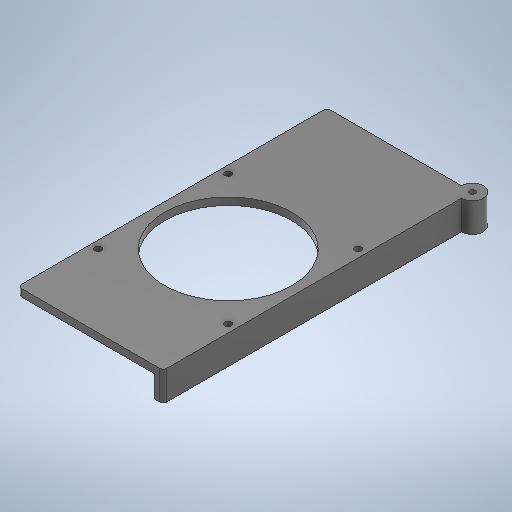
# Autodesk Inventor part: Power Box (12V) Cover
Saved by Autodesk Inventor 2026.2 (Build 302298010, 298A)
## iProperties
Created: 2026-05-26
Part Number: Power Box (12V) Cover
Material: ABS Plastic
Document SubType Name: Modeling
Designer: chanh
Density: 1.06 g/cm^3
Appearance: Smooth - White
Author: chanh
Autodesk Inventor part; units mm, degrees
ref_plane "YZ Plane" through (0, 0, 0) normal (1, 0, 0) x (0, 1, 0)
ref_plane "XZ Plane" through (0, 0, 0) normal (0, 1, 0) x (-1, 0, 0)
ref_plane "XY Plane" through (0, 0, 0) normal (0, 0, 1) x (1, 0, 0)
sketch "Sketch1" plane through (0, 0, 0) normal (0, 1, 0) x (-1, 0, 0)
  line L0 (40, 85) -> (-40, 85)
  line L1 (-40, 85) -> (-40, -85)
  line L2 (-40, -85) -> (40, -85)
  line L3 (40, -85) -> (40, 85)
  line L4 (40, 85) -> (-40, -85) construction
  line L5 (-40, 85) -> (40, -85) construction
  circle A0 centre (-40, -85) radius 6
  point P0 (0, 0)
  point P1 (-40, -79)
  point P2 (-34, -85)
  dimension "d0" = 80
  dimension "d1" = 170
  dimension "d2" = 12
  constraints: 12 end point, 2 midpoint, 2 parallel, 1 centre point, 1 coincident, 1 horizontal, 1 perpendicular
  measures "d0" distance of L2.end L1.end
  measures "d1" distance of L0.end L1.end
  measures "d2" diameter of A0
extrude "Extrusion1" add sketch "Sketch1" along normal blind 4
sketch "Sketch2" plane through (0, 0, 0) normal (0, -1, 0) x (1, 0, 0)
  line L0 (40, 85) -> (40, -79) projected
  line L1 (-40, 85) -> (40, 85) projected
  line L2 (-40, -85) -> (-40, 85) projected
  line L3 (34, -85) -> (-40, -85) projected
  arc A0 (34, -85) -> (40, -79) centre (40, -85) ccw projected
  line L4 (35, 85) -> (35, -80)
  line L5 (35, -80) -> (-40, -80)
  point P0 (0, 0)
  dimension "d5" = 5
  dimension "d6" = 5
  constraints: 4 end point, 2 point on line, 1 perpendicular, 1 vertical
  measures "d5" distance between parallel lines of L3 L5
  measures "d6" distance between parallel lines of L0 L4
extrude "Extrusion2" add sketch "Sketch2" along normal blind 12 contours L0 A0 L3 L2 L5 L4 L1
sketch "Sketch3" plane through (0, 4, 0) normal (0, 1, 0) x (1, 0, 0)
  arc A0 (40, 79) -> (34, 85) centre (40, 85) ccw projected
  arc A1 (40, 79) -> (34, 85) centre (40, 85) ccw projected
  point P0 (0, 0)
hole "Hole1" at (40, 4, -85) direction (0, -1, 0) diameter 3.2 end through all
sketch "Sketch4" plane through (0, 4, 0) normal (0, 1, 0) x (1, 0, 0)
  line L0 (35.75, -45) -> (-35.75, -45) construction
  line L1 (-35.75, -45) -> (-35.75, 26.5) construction
  line L2 (-35.75, 26.5) -> (35.75, 26.5) construction
  line L3 (35.75, 26.5) -> (35.75, -45) construction
  line L4 (35.75, -45) -> (-35.75, 26.5) construction
  line L5 (-35.75, -45) -> (35.75, 26.5) construction
  circle A0 centre (40, 85) radius 1.6 projected
  line L6 (40, -85) -> (40, 79) projected
  arc A1 (40, 79) -> (34, 85) centre (40, 85) ccw projected
  line L7 (34, 85) -> (-40, 85) projected
  line L8 (-40, 85) -> (-40, -85) projected
  line L9 (-40, -85) -> (40, -85) projected
  point P0 (0, 0)
  point P1 (0, -9.25)
  dimension "d16" = 71.5
  dimension "d17" = 40
  constraints: 12 end point, 4 coincident, 2 midpoint, 2 parallel, 2 perpendicular, 1 horizontal, 1 vertical alignment
  measures "d16" distance of L0.end L1.end
  measures "d17" distance between parallel lines of L9 L0
hole "Hole2" at (-35.75, 4, 45) at (-35.75, 4, -26.5) at (35.75, 4, 45) at (35.75, 4, -26.5) direction (0, -1, 0) diameter 3.7 end through all
sketch "Sketch5" plane through (0, 4, 0) normal (0, 1, 0) x (1, 0, 0)
  circle A0 centre (0, -9.25) radius 35
  point P0 (0, 0)
  point P1 (0, -9.25)
  dimension "d25" = 70
  constraints: 1 centre point, 1 coincident
  measures "d25" diameter of A0
extrude "Extrusion3" cut sketch "Sketch5" against normal up to surface (4 mm away)
fillet "Fillet1" radius 2 3 edges at (-40, -4, -85) (-40, 2, 85) (40, -4, 85)
equation "\"d6\" = d5"
body "Solid1"
